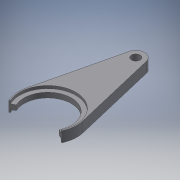
# Autodesk Inventor part: fork
Saved by Autodesk Inventor 2017 (Build 210142000, 142)
## iProperties
Created: 2018-04-16
Part Number: fork
Material: Generic
Document SubType Name: Modeling
Designer: RKL
Density: 1 g/cm^3
Appearance: Default
Author: RKL
Autodesk Inventor part; units mm, degrees
ref_plane "YZ Plane" through (0, 0, 0) normal (1, 0, 0) x (0, 1, 0)
ref_plane "XZ Plane" through (0, 0, 0) normal (0, 1, 0) x (-1, 0, 0)
sketch "Sketch1" plane through (0, 0, 0) normal (0, 0, 1) x (1, 0, 0)
  circle A0 centre (0, 0) radius 21.5
  arc A1 (-25.7817, 6.1281) -> (25.7817, 6.1281) centre (0, 0) ccw
  line L0 (0, 0) -> (0, 80) construction
  circle A2 centre (0, 80) radius 4
  arc A3 (7.7832, 81.85) -> (-7.7832, 81.85) centre (0, 80) ccw
  line L1 (-7.7832, 81.85) -> (-25.7817, 6.1281)
  line L2 (7.7832, 81.85) -> (25.7817, 6.1281)
  dimension "d0" = 43
  dimension "d1" = 8
  dimension "d2" = 80
  dimension "d3" = 8
  dimension "d4" = 5
  constraints: 6 end point, 4 centre point, 4 coincident, 4 point on circle, 4 tangent, 1 vertical
  measures "d0" diameter of A0
  measures "d1" diameter of A2
  measures "d2" distance of L0.start L0.end
  measures "d3" radius of A3
  measures "d4" radial gap between concentric circles of A0 A1
extrude "Extrusion1" add sketch "Sketch1" along normal blind 4.5
sketch "Sketch2" plane through (0, 0, 4.5) normal (0, 0, 1) x (1, 0, 0)
  circle A0 centre (0, 0) radius 21.5 projected
  circle A1 centre (0, 80) radius 4 projected
  arc A2 (-25.7817, 6.1281) -> (25.7817, 6.1281) centre (0, 0) ccw projected
  line L0 (25.7817, 6.1281) -> (7.7832, 81.85) projected
  arc A3 (7.7832, 81.85) -> (-7.7832, 81.85) centre (0, 80) ccw projected
  line L1 (-7.7832, 81.85) -> (-25.7817, 6.1281) projected
  circle A4 centre (0, 0) radius 25.5
  dimension "d7" = 51
  constraints: 1 centre point, 1 coincident
  measures "d7" diameter of A4
extrude "Extrusion2" add sketch "Sketch2" along normal blind 2.5 contours L1 A3 L0 A2
ref_plane "Work Plane1" through (0, 0, 2.25) normal (0, 0, 1) x (1, 0, 0)
mirror "Mirror1" about plane through (0, 0, 2.25) normal (0, 0, 1) of "Extrusion2"
sketch "Sketch3" plane through (0, 0, 7) normal (0, 0, 1) x (1, 0, 0)
  arc A0 (-25.7817, 6.1281) -> (25.7817, 6.1281) centre (0, 0) ccw construction
  line L0 (0, 0) -> (-24.0172, -11.1994)
  line L1 (0, 0) -> (24.0172, -11.1994)
  arc A1 (-24.0172, -11.1994) -> (24.0172, -11.1994) centre (0, 0) ccw
  line L2 (0, 0) -> (0, -26.5) construction
  dimension "d10" = 130
  constraints: 6 end point, 5 point on circle, 1 centre point, 1 coincident, 1 concentric, 1 vertical
  measures "d10" angle of L1 L0
extrude "Extrusion3" cut sketch "Sketch3" against normal through all
body "Solid1"
